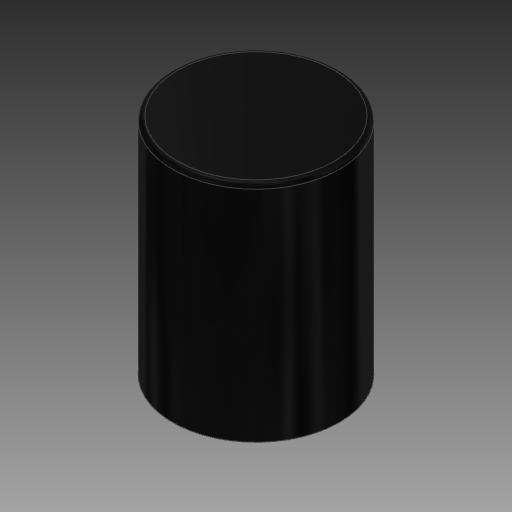
# Autodesk Inventor part: Kondensator 30x50
Saved by Autodesk Inventor 2019.4 (Build 234330000, 330)
## iProperties
Created: 2012-08-01
Part Number: Kondensator 30x50
Material: PC/ABS-Kunststoff
Document SubType Name: Modeling
Designer: rYan
Density: 1.493 g/cm^3
Mass: 67.5152 g
Surface Area: 70.9477 cm^2
Volume: 45.2211 cm^3
Appearance: Glänzend - schwarz
Author: rYan
Autodesk Inventor part; units mm, degrees
ref_plane "YZ Plane" through (0, 0, 0) normal (1, 0, 0) x (0, 1, 0)
ref_plane "XY Plane" through (0, 0, 0) normal (0, 0, 1) x (1, 0, 0)
sketch "Skizze1" plane through (0, 0, 0) normal (0, 0, 1) x (1, 0, 0)
  circle A0 centre (0, 0) radius 17.5
  dimension "d0" = 35
  constraints: 1 centre point, 1 coincident
  measures "d0" diameter of A0
extrude "Extrusion1" add sketch "Skizze1" along normal blind 47
fillet "Rundung1" radius 1 1 edges at (-17.5, 0, 47)
sketch "Skizze2" plane through (0, 0, 0) normal (0, 0, -1) x (-1, 0, 0)
  line L0 (-24.5, 0) -> (24.5, 0) projected
  line L1 (0, -24.5) -> (0, 24.5) projected
  circle A0 centre (-5, 0) radius 1
  circle A1 centre (5, 0) radius 1
  dimension "d4" = 10
  dimension "d5" = 2
  constraints: 2 centre point, 2 coincident, 2 point on line, 1 symmetric about line, 1 other
  measures "d4" distance of point (5, 0) point (-5, 0)
  measures "d5" diameter of A0
extrude "Extrusion2" add sketch "Skizze2" along normal blind 4
ref_plane "Arbeitsebene1" through (0, 0, 0) normal (0, 1, 0) x (-1, 0, 0)
